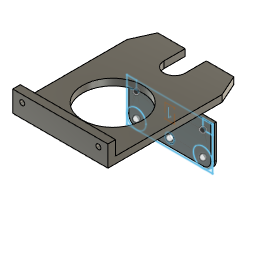
Spool Side (Autodesk Fusion 360 design; units mm, degrees)
Autodesk Fusion 360 part; units mm, degrees
note: some values were not read from the file. Set by a fixed rule: which sketch regions a step uses.
sketch "Sketch1" plane through (0, 0, 0) normal (0, 0, 1) x (1, 0, 0)
  circle A0 centre (0, 0) radius 11.125
  line L0 (-11.125, 0) -> (11.125, 0)
  line L1 (11.125, 0) -> (11.125, 22.25)
  line L2 (11.125, 22.25) -> (-11.125, 22.25)
  line L3 (-11.125, 22.25) -> (-11.125, 0)
  line L4 (40, 22.25) -> (-40, 22.25)
  line L5 (-40, 22.25) -> (-40, -22.25)
  line L6 (-40, -22.25) -> (40, -22.25)
  line L7 (40, -22.25) -> (40, 22.25)
  line L8 (40, 22.25) -> (-40, -22.25) construction
  line L9 (-40, 22.25) -> (40, -22.25) construction
  line L10 (0, 0) -> (-50, 0)
  line L11 (-50, 0) -> (-50, -120)
  line L12 (-50, -120) -> (0, -120)
  line L13 (0, -120) -> (0, 0)
  line L14 (0, 0) -> (50, 0)
  line L15 (50, 0) -> (50, -120)
  line L16 (50, -120) -> (0, -120)
  line L17 (0, -120) -> (0, 0)
  line L18 (-40, 22.25) -> (-50, 0)
  line L19 (40, 22.25) -> (50, 0)
  circle A1 centre (0, -65) radius 31.6228
  dimension "d1" = 22.25
  dimension "d2" = 22.25
  dimension "d3" = 22.25
  dimension "d4" = 80
  dimension "d5" = 44.5
  dimension "d7" = 50
  dimension "d8" = 120
  constraint coincident A0.centre L10.start
  constraint horizontal L0
  constraint vertical L1
  constraint horizontal L2
  constraint vertical L3
  constraint coincident A0 L0.start
  constraint horizontal L4
  constraint perpendicular L4 L5
  constraint parallel L4 L6
  constraint parallel L5 L7
  constraint coincident L8 A0.centre
  constraint coincident L9 A0.centre
  constraint horizontal L10
  constraint vertical L11
  constraint horizontal L12
  constraint vertical L13
  constraint horizontal L14
  constraint vertical L15
  constraint horizontal L16
  constraint vertical L17
  constraint coincident L17 A1.centre
  measures "d1" diameter of A0
  measures "d2" distance of L0.start L0.end
  measures "d3" distance of L0.start L2.end
  measures "d4" distance of L5.end L6.end
  measures "d5" distance of L4.end L5.end
  measures "d7" distance of A0.centre L10.end
  measures "d8" distance of A0.centre L12.end
extrude "Extrude1" add sketch "Sketch1" along normal blind 7 contours A0 L6 L7 L13 L14 L17 | L1 L4 L7 L14 | L3 L4 L5 L10 | A0 L5 L6 L10 L13 L17 | L6 L7 L13 L14 L15 L16 L17 A1 | L7 L14 L19 | L5 L10 L18 | L5 L6 L10 L11 L12 L13 L17 A1 makes body 1
sketch "Sketch2" plane through (0, 0, 7) normal (0, 0, 1) x (-1, 0, 0)
  circle A0 centre (0, 65) radius 31.6228
  line L0 (11.125, -22.25) -> (40, -22.25)
  line L1 (40, -22.25) -> (50, 0)
  line L2 (50, 0) -> (50, 120)
  line L3 (50, 120) -> (-50, 120)
  line L4 (-50, 120) -> (-50, 0)
  line L5 (-50, 0) -> (-40, -22.25)
  line L6 (-40, -22.25) -> (-11.125, -22.25)
  line L7 (-11.125, -22.25) -> (-11.125, 0)
  arc A1 (11.125, 0) -> (-11.125, 0) centre (0, 0) ccw
  line L8 (11.125, 0) -> (11.125, -22.25)
  line L9 (50, 120) -> (-50, 120)
  line L10 (-50, 120) -> (-50, 112)
  line L11 (-50, 112) -> (50, 112)
  line L12 (50, 112) -> (50, 120)
  dimension "d11" = 100
  dimension "d12" = 8
  constraint horizontal L9
  constraint vertical L10
  constraint horizontal L11
  constraint vertical L12
  constraint coincident L2.end L3.start
  measures "d11" distance of L2.end L3.end
  measures "d12" distance of L2.end L11.end
extrude "Extrude2" add sketch "Sketch2" along normal blind 15 contours L2 L3 L4 L9 L10 L11 L12 bodies 1
sketch "Sketch3" plane through (0, -112, 0) normal (0, 1, 0) x (-1, 0, 0)
  line L0 (-50, 7) -> (50, 7)
  line L1 (50, 7) -> (50, 22)
  line L2 (50, 22) -> (-50, 22)
  line L3 (-50, 22) -> (-50, 7)
  line L4 (-50, 22) -> (50, 22)
  line L5 (50, 22) -> (50, 14.5)
  line L6 (50, 14.5) -> (-50, 14.5)
  line L7 (-50, 14.5) -> (-50, 22)
  line L8 (-50, 22) -> (-40, 22)
  line L9 (-40, 22) -> (-40, 14.5)
  line L10 (-40, 14.5) -> (-50, 14.5)
  line L11 (-50, 14.5) -> (-50, 22)
  line L12 (50, 22) -> (40, 22)
  line L13 (40, 22) -> (40, 14.5)
  line L14 (40, 14.5) -> (50, 14.5)
  line L15 (50, 14.5) -> (50, 22)
  circle A0 centre (-40, 14.5) radius 2.625
  circle A1 centre (40, 14.5) radius 2.625
  dimension "d15" = 100
  dimension "d16" = 7.5
  dimension "d17" = 10
  dimension "d18" = 10
  dimension "d19" = 5.25
  dimension "d20" = 5.25
  constraint horizontal L4
  constraint vertical L5
  constraint horizontal L6
  constraint vertical L7
  constraint coincident L2.end L3.start
  constraint horizontal L8
  constraint vertical L9
  constraint horizontal L10
  constraint vertical L11
  constraint coincident L6 L9.end
  constraint horizontal L12
  constraint vertical L13
  constraint horizontal L14
  constraint vertical L15
  constraint coincident L1.end L2.start
  constraint coincident L9.end L10.start
  constraint coincident L13.end L14.start
  measures "d15" distance of L2.end L1.end
  measures "d16" distance of L2.end L6.end
  measures "d17" distance of L2.end L8.end
  measures "d18" distance of L1.end L12.end
  measures "d19" diameter of A0
  measures "d20" diameter of A1
extrude "Extrude3" cut sketch "Sketch3" against normal blind 9 contours L6 L9 L10 A0 | L6 L10 A0 | L6 L14 A1 | L6 L13 L14 A1 | L6 L9 A0 | L6 L13 A1 bodies 1
sketch "Sketch1 (2)" plane through (0, 0, 0) normal (0, 1, 0) x (1, 0, 0) in component "Front Bowden Holder"
  line L0 (-50, 25) -> (40, 25)
  line L1 (40, 25) -> (40, 70)
  line L2 (40, 70) -> (-50, 70)
  line L3 (-50, 70) -> (-50, 25)
  circle A0 centre (-40, 60) radius 10
  circle A1 centre (30, 60) radius 10
  circle A2 centre (-5, 60) radius 4.7
  line L4 (-50, 25) -> (-40, 25)
  line L5 (-40, 25) -> (-40, 35)
  line L6 (-40, 35) -> (-50, 35)
  line L7 (-50, 35) -> (-50, 25)
  line L8 (40, 25) -> (30, 25)
  line L9 (30, 25) -> (30, 35)
  line L10 (30, 35) -> (40, 35)
  line L11 (40, 35) -> (40, 25)
  circle A3 centre (-40, 35) radius 1.75
  circle A4 centre (30, 35) radius 1.75
  line L12 (0, 30) -> (-10, 30) construction
  line L13 (-10, 30) -> (-10, 45) construction
  line L14 (-10, 45) -> (0, 45) construction
  line L15 (0, 45) -> (0, 30) construction
  dimension "d23" = 90
  dimension "d24" = 45
  dimension "d25" = 10
  dimension "d26" = 10
  dimension "d27" = 9.4
  dimension "d32" = 3.5
  dimension "d33" = 3.5
  dimension "d36" = 10
  text T0 "1" font "Arial" height 10 align centre middle in box 10 x 15 at (0, 30) x (-1, 0) y (0, 1) spacing 1
  constraint horizontal L0
  constraint vertical L1
  constraint horizontal L2
  constraint vertical L3
  constraint tangent L3 A0
  constraint tangent L2 A0
  constraint tangent L2 A1
  constraint tangent L1 A1
  constraint horizontal L4
  constraint vertical L5
  constraint horizontal L6
  constraint vertical L7
  constraint horizontal L8
  constraint vertical L9
  constraint horizontal L10
  constraint vertical L11
  constraint coincident L5.end L6.start
  constraint coincident L9.end L10.start
  measures "d23" distance of L0.start L0.end
  measures "d24" distance of L0.start L2.end
  measures "d25" radius of A0
  measures "d26" radius of A1
  measures "d27" diameter of A2
  measures "d32" diameter of A3
  measures "d33" diameter of A4
extrude "Extrude1'" add sketch "Sketch1 (2)" along normal blind 4 separate body contours L0 L3 L4 L5 L6 L7 A3 | L0 L1 L2 L3 A0 A1 L5 L6 L9 L10 A3 A4 | L0 L1 L8 L9 L10 L11 A4 | L5 L6 A3 | L5 L6 A3 | A0 | L9 L10 A4 | L9 L10 A4 | A1 makes body 2 in component "Front Bowden Holder"
fillet "Fillet1" radius 2 5 edges at (40, 0, -42.5) (37.0711, 0, -67.0711) (-5, 0, -70) (-47.0711, 0, -67.0711) (-50, 0, -42.5) on bodies 2 in component "Front Bowden Holder"
extrude "Extrude2'" cut sketch "Sketch1 (2)" along normal blind 29.794 contours L5 L6 A3 | L5 L6 A3 | L9 L10 A4 | L9 L10 A4 bodies 2 in component "Front Bowden Holder"
extrude "Extrude3'" add sketch "Sketch1 (2)" against normal blind 1 text T0 bodies 2 in component "Front Bowden Holder"
component "Front Bowden Holder" placed x (1, 0, 0) y (0, 1, 0) z (0, 0, 1) at (0, 0, 0)
